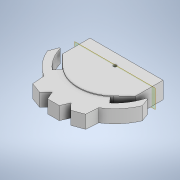
# Autodesk Inventor part: Деталь3
Saved by Autodesk Inventor 2020 (Build 240168000, 168)
## iProperties
Created: 2022-06-10
Part Number: Деталь3
Material: Типовые
Document SubType Name: Modeling
Designer: NoName
Density: 1 g/cm^3
Appearance: По умолчанию
Author: NoName
Autodesk Inventor part; units mm, degrees
ref_plane "YZ Plane" through (0, 0, 0) normal (1, 0, 0) x (0, 1, 0)
ref_plane "XZ Plane" through (0, 0, 0) normal (0, 1, 0) x (-1, 0, 0)
ref_plane "XY Plane" through (0, 0, 0) normal (0, 0, 1) x (1, 0, 0)
sketch "Эскиз3" plane through (0, 0, 0) normal (0, 1, 0) x (-1, 0, 0)
  arc A0 (3.3164, 4.9701) -> (-3.3164, 4.9701) centre (0, 1.5) ccw
  line L0 (-4.75, 0) -> (-4.75, 3.6)
  line L1 (-4.75, 3.6) -> (-3.3164, 4.9701)
  line L2 (-4.75, 0) -> (4.75, 0)
  line L3 (0, 0) -> (0, 6.3)
  line L4 (4.75, 0) -> (4.75, 3.6)
  line L5 (4.75, 3.6) -> (3.3164, 4.9701)
  dimension "d36" = 4.8
  dimension "d38" = 9.5
  dimension "d39" = 3.6
  dimension "d40" = 1.5
  constraints: 12 end point, 3 point on circle, 2 vertical, 1 centre point, 1 coincident, 1 horizontal, 1 horizontal alignment, 1 midpoint, 1 symmetric about line, 1 tangent, 1 vertical alignment
  measures "d36" radius of A0
  measures "d38" distance between parallel lines of L4 L0
  measures "d39" distance from line of L0.end L2
  measures "d40" distance from line of L2 A0.centre
extrude "Выдавливание1" add sketch "Эскиз3" along normal blind 0.4
sketch "Эскиз4" plane through (0, 0.4, 0) normal (0, 1, 0) x (1, 0, 0)
  line L0 (-4.75, 0) -> (-4.75, -3.6) projected
  line L1 (-4.75, -3.6) -> (-3.3164, -4.9701) projected
  arc A0 (-3.3164, -4.9701) -> (3.3164, -4.9701) centre (0, -1.5) ccw projected
  line L2 (3.3164, -4.9701) -> (4.75, -3.6) projected
  line L3 (4.75, -3.6) -> (4.75, 0) projected
  line L4 (4.75, 0) -> (-4.75, 0) projected
  arc A1 (-3.3164, -4.9701) -> (3.3164, -4.9701) centre (0, -1.5) ccw projected
  line L5 (-1.6417, -6.0105) -> (-1.9837, -6.9502)
  arc A2 (-4.7186, -4.8726) -> (-1.9837, -6.9502) centre (0, -1.5) ccw
  line L6 (-4.9, -4.9307) -> (-4.9, -6.0695)
  arc A3 (-4.9, -6.0695) -> (-1.4, -8.0521) centre (0, -1.5) ccw
  line L7 (-1.4, -8.0521) -> (-0.75, -9.5)
  line L8 (-0.75, -9.5) -> (0, -9.5)
  line L9 (0, -9.5) -> (0, 0)
  arc A4 (-1.6417, -6.0105) -> (0, -6.3) centre (0, -1.5) ccw
  arc A5 (-4.7186, -4.8726) -> (-4.9, -4.9307) centre (-4.8, -4.9307) ccw
  line L10 (1.6417, -6.0105) -> (1.9837, -6.9502)
  arc A6 (1.9837, -6.9502) -> (4.7186, -4.8726) centre (0, -1.5) ccw
  line L11 (4.9, -4.9307) -> (4.9, -6.0695)
  arc A7 (1.4, -8.0521) -> (4.9, -6.0695) centre (0, -1.5) ccw
  line L12 (1.4, -8.0521) -> (0.75, -9.5)
  line L13 (0.75, -9.5) -> (0, -9.5)
  arc A8 (0, -6.3) -> (1.6417, -6.0105) centre (0, -1.5) ccw
  arc A9 (4.9, -4.9307) -> (4.7186, -4.8726) centre (4.8, -4.9307) ccw
  point P0 (-4.9, -4.6032)
  dimension "d81" = 0.1
  dimension "d82" = 9.8
  dimension "d83" = 5.8
  dimension "d84" = 6.7
  dimension "d85" = 9.5
  dimension "d86" = 2.8
  dimension "d87" = 1.5
  dimension "d88" = 40
  constraints: 19 point on circle, 18 end point, 8 centre point, 8 symmetric about line, 3 coincident, 2 point on line, 2 tangent, 2 vertical, 1 horizontal, 1 line through centre, 4 other
  measures "d81" radius of A5
  measures "d82" distance between parallel lines of L11 L6
  measures "d83" radius of A2
  measures "d84" radius of A3
  measures "d85" distance between parallel lines of L4 L8
  measures "d86" distance of L12.start L7.start
  measures "d87" distance of L12.end L7.end
  measures "d88" angle of L10 L5
extrude "Выдавливание2" add sketch "Эскиз4" along normal blind 1.7 contours L9 L8 L7 A3 L6 A5 A2 L5 A0 | A0 L10 A6 A9 L11 A7 L12 L13 L9
sketch "Эскиз9" plane through (0, 0.4, 0) normal (0, 1, 0) x (1, 0, 0)
  line L0 (-4.75, 0) -> (-4.75, -3.6) projected
  line L1 (-4.75, -3.6) -> (-3.3164, -4.9701) projected
  arc A0 (-3.3164, -4.9701) -> (-1.6417, -6.0105) centre (0, -1.5) ccw projected
  arc A1 (-1.6417, -6.0105) -> (1.6417, -6.0105) centre (0, -1.5) ccw projected
  arc A2 (1.6417, -6.0105) -> (3.3164, -4.9701) centre (0, -1.5) ccw projected
  line L2 (3.3164, -4.9701) -> (4.75, -3.6) projected
  line L3 (4.75, -3.6) -> (4.75, 0) projected
  line L4 (4.75, 0) -> (-4.75, 0) projected
  point P0 (0, 0)
extrude "Выдавливание4" add sketch "Эскиз9" along normal blind 1.8
ref_plane "РабПлоскость2" through (4.75, 0, 1.5) normal (0, 0, -1) x (-1, 0, 0)
sketch "Эскиз10" plane through (4.75, 0, 1.5) normal (0, 0, -1) x (-1, 0, 0)
  line L0 (4.75, 0) -> (4.75, 2.2)
  line L1 (0, 2.2) -> (9.5, 2.2) projected
  line L2 (8.0664, 2.2) -> (1.4336, 2.2) projected
  line L3 (4.75, 0) -> (4.95, 0)
  line L4 (4.95, 0) -> (4.95, 2.2)
  line L5 (4.95, 2.2) -> (4.75, 2.2)
  line L6 (4.75, 2.2) -> (4.75, 0)
  dimension "d98" = 0.4
  constraints: 10 end point, 2 parallel, 1 horizontal, 1 midpoint, 1 perpendicular, 1 point on line
  measures "d98" diameter of L4 L0
revolve "Вращение1" cut sketch "Эскиз10" angle 360 about axis through (0, 0, 1.5) along (0, 1, 0)
pattern_circular "Круговой массив1" count 3 over 40 about axis through (0, 1.1, 1.5) along (0, 1, 0) of "Выдавливание2" both ways yes
